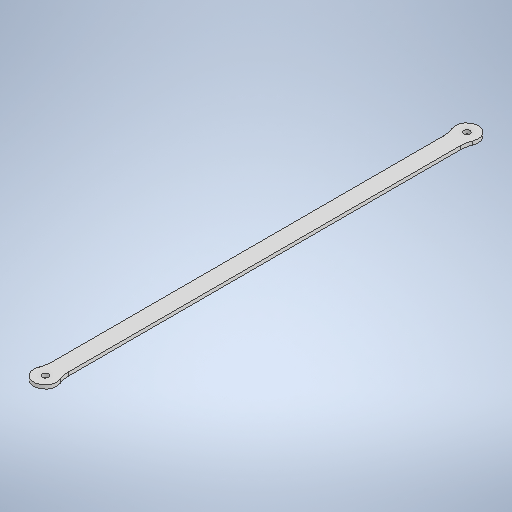
# Autodesk Inventor part: A2P1
Saved by Autodesk Inventor 2025.2 (Build 292293000, 293)
## iProperties
Created: 2025-05-22
Part Number: A2P1
Material: Generic
Document SubType Name: Sheet Metal
Designer: Admin
Density: 1 g/cm^3
Sheet Metal Rule: Default
Appearance: Default
Author: Admin
Autodesk Inventor part; units mm, degrees
ref_plane "YZ Plane" through (0, 0, 0) normal (1, 0, 0) x (0, 1, 0)
ref_plane "XZ Plane" through (0, 0, 0) normal (0, 1, 0) x (-1, 0, 0)
ref_plane "XY Plane" through (0, 0, 0) normal (0, 0, 1) x (1, 0, 0)
sketch "Sketch1" plane through (0, 0, 0) normal (0, 1, 0) x (-1, 0, 0)
  arc A0 (5.0015, -2.165) -> (-5.0015, -2.165) centre (0, 0) ccw
  line L0 (4, -7) -> (4, -193)
  line L1 (-4, -7) -> (-4, -193)
  arc A1 (5.0015, -2.165) -> (4, -7) centre (16.1716, -7) ccw
  arc A2 (-4, -7) -> (-5.0015, -2.165) centre (-16.1716, -7) ccw
  arc A3 (-5.0015, -197.835) -> (5.0015, -197.835) centre (0, -200) ccw
  arc A4 (4, -193) -> (5.0015, -197.835) centre (16.1716, -193) ccw
  arc A5 (-5.0015, -197.835) -> (-4, -193) centre (-16.1716, -193) ccw
  dimension "d0" = 10.9
  dimension "d4" = 4
  dimension "d5" = 4
  dimension "d6" = 0
  dimension "d7" = 10.9
  dimension "d8" = 200
  dimension "d9" = 0
  dimension "d10" = 7
  dimension "d12" = 4
  dimension "d13" = 7
  constraints: 14 point on circle, 8 tangent, 6 centre point, 4 end point, 2 vertical, 1 coincident
  measures "d0" diameter of A0
  measures "d4" horizontal distance of point (0, 0) L0.start
  measures "d5" horizontal distance of point (0, 0) L1.start
  measures "d6" vertical distance of L0.start L1.start
  measures "d7" diameter of A3
  measures "d8" distance of A3.centre point (0, 0)
  measures "d9" vertical distance of A5.centre L0.end
  measures "d10" vertical distance of L0.start point (0, 0)
  measures "d12" horizontal distance of A3.centre L0.end
  measures "d13" vertical distance of A3.centre L0.end
extrude "Extrusion1" add sketch "Sketch1" along normal blind 1.7
sketch "Sketch2" plane through (0, 1.7, 0) normal (0, 1, 0) x (1, 0, 0)
  arc A0 (5.0015, 197.835) -> (-5.0015, 197.835) centre (0, 200) ccw projected
  arc A1 (-5.0015, 2.165) -> (5.0015, 2.165) centre (0, 0) ccw projected
  circle A2 centre (0, 0) radius 1.5
  circle A3 centre (0, 200) radius 1.5
  dimension "d16" = 3
  dimension "d17" = 3
  constraints: 2 centre point, 2 coincident
  measures "d16" diameter of A3
  measures "d17" diameter of A2
extrude "Extrusion2" cut sketch "Sketch2" against normal blind 1.7
equation "\"BendRadius\" = Thickness"
equation "\"BendReliefWidth\" = Thickness"
equation "\"BendReliefDepth\" = 0.5 * Thickness"
equation "\"CornerReliefSize\" = 4 * Thickness"
equation "\"MinimumRemnant\" = 2 * Thickness"
equation "\"TransitionRadius\" = BendRadius"
equation "\"JacobiRadiusSize\" = BendRadius"
equation "\"GapSize\" = Thickness"
equation "\"Thickness\" = 3.048"
body "Solid1"
